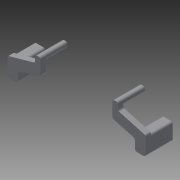
# Autodesk Inventor part: Solenoid Mount
Saved by Autodesk Inventor 2015 (Build 190159000, 159)
## iProperties
Created: 2016-09-23
Part Number: Solenoid Mount
Material: Generic
Document SubType Name: Modeling
Designer: James Yelland
Density: 1 g/cm^3
Appearance: Default
Author: James Yelland
Autodesk Inventor part; units mm, degrees
ref_plane "YZ Plane" through (0, 0, 0) normal (1, 0, 0) x (0, 1, 0)
ref_plane "XZ Plane" through (0, 0, 0) normal (0, 1, 0) x (-1, 0, 0)
ref_plane "XY Plane" through (0, 0, 0) normal (0, 0, 1) x (1, 0, 0)
sketch "Sketch1" plane through (0, 0, 0) normal (0, 1, 0) x (-1, 0, 0)
  line L0 (-54.0074, -78) -> (-54.0074, -71.5202)
  arc A0 (-52.5426, -69.5932) -> (-54.0074, -71.5202) centre (-52.0074, -71.5202) ccw
  arc A1 (-56.0074, -80) -> (-54.0074, -78) centre (-56.0074, -78) ccw
  line L1 (-54.0074, -78) -> (-54.0074, -71.5202)
  arc A2 (-52.5426, -69.5932) -> (-54.0074, -71.5202) centre (-52.0074, -71.5202) ccw
  arc A3 (-56.0074, -80) -> (-54.0074, -78) centre (-56.0074, -78) ccw
  line L2 (-54.0074, -78) -> (-54.0074, -71.5202)
  arc A4 (-52.5426, -69.5932) -> (-54.0074, -71.5202) centre (-52.0074, -71.5202) ccw
  arc A5 (-56.0074, -80) -> (-54.0074, -78) centre (-56.0074, -78) ccw
  line L3 (-62.0074, -80) -> (-56.0074, -80)
  line L4 (-64.0074, -78) -> (-64.0074, -64.2976)
  arc A6 (-62.5426, -62.3706) -> (-64.0074, -64.2976) centre (-62.0074, -64.2976) ccw
  arc A7 (-64.0074, -78) -> (-62.0074, -80) centre (-62.0074, -78) ccw
  line L5 (-52.5426, -69.5932) -> (-34.7368, -64.6478)
  line L6 (-33.272, -62.7207) -> (-33.272, -56.3381)
  line L7 (-33.272, -56.3381) -> (-33.272, -54)
  line L8 (-33.272, -54) -> (-33.272, -51)
  line L9 (-35.272, -49) -> (-36.272, -49)
  line L10 (-62.5426, -62.3706) -> (-39.7368, -56.0365)
  line L11 (-38.272, -54.1094) -> (-38.272, -51)
  arc A8 (-36.272, -49) -> (-38.272, -51) centre (-36.272, -51) ccw
  arc A9 (-33.272, -51) -> (-35.272, -49) centre (-35.272, -51) ccw
  arc A10 (-39.7368, -56.0365) -> (-38.272, -54.1094) centre (-40.272, -54.1094) ccw
  arc A11 (-34.7368, -64.6478) -> (-33.272, -62.7207) centre (-35.272, -62.7207) ccw
  line L12 (54.0074, -78) -> (54.0074, -71.5202)
  arc A12 (54.0074, -71.5202) -> (52.5426, -69.5932) centre (52.0074, -71.5202) ccw
  arc A13 (54.0074, -78) -> (56.0074, -80) centre (56.0074, -78) ccw
  line L13 (54.0074, -78) -> (54.0074, -71.5202)
  arc A14 (54.0074, -71.5202) -> (52.5426, -69.5932) centre (52.0074, -71.5202) ccw
  arc A15 (54.0074, -78) -> (56.0074, -80) centre (56.0074, -78) ccw
  line L14 (54.0074, -78) -> (54.0074, -71.5202)
  arc A16 (54.0074, -78) -> (56.0074, -80) centre (56.0074, -78) ccw
  arc A17 (54.0074, -71.5202) -> (52.5426, -69.5932) centre (52.0074, -71.5202) ccw
  line L15 (62.0074, -80) -> (56.0074, -80)
  line L16 (64.0074, -78) -> (64.0074, -64.2976)
  arc A18 (64.0074, -64.2976) -> (62.5426, -62.3706) centre (62.0074, -64.2976) ccw
  arc A19 (62.0074, -80) -> (64.0074, -78) centre (62.0074, -78) ccw
  line L17 (52.5426, -69.5932) -> (34.7368, -64.6478)
  line L18 (33.272, -62.7207) -> (33.272, -56.3381)
  line L19 (33.272, -56.3381) -> (33.272, -54)
  line L20 (33.272, -54) -> (33.272, -51)
  line L21 (35.272, -49) -> (36.272, -49)
  line L22 (62.5426, -62.3706) -> (39.7368, -56.0365)
  line L23 (38.272, -54.1094) -> (38.272, -51)
  arc A20 (38.272, -51) -> (36.272, -49) centre (36.272, -51) ccw
  arc A21 (35.272, -49) -> (33.272, -51) centre (35.272, -51) ccw
  arc A22 (38.272, -54.1094) -> (39.7368, -56.0365) centre (40.272, -54.1094) ccw
  arc A23 (33.272, -62.7207) -> (34.7368, -64.6478) centre (35.272, -62.7207) ccw
  point P0 (-33.272, -64.241)
  point P1 (-33.272, -49)
  point P2 (-38.272, -49)
  point P3 (33.272, -64.241)
  point P4 (33.272, -49)
  point P5 (38.272, -49)
  dimension "d11" = 2
  dimension "d29" = 20
  dimension "d30" = 5
  dimension "d31" = 5
  dimension "d32" = 2
  constraints: 48 end point, 48 point on circle, 24 centre point, 16 point on line, 13 tangent, 4 equal radius, 2 perpendicular, 1 vertical
  measures "d11" radius of A6
  measures "d29" distance of L5.start point (-33.272, -64.241)
  measures "d30" distance of L7.end point (-33.272, -49)
  measures "d31" distance of point (-33.272, -49) point (-38.272, -49)
  measures "d32" radius of A8
extrude "Extrusion1" add sketch "Sketch1" along normal blind 5
sketch "Sketch2" plane through (0, 5, 0) normal (0, 1, 0) x (1, 0, 0)
  line L0 (54.0074, 78) -> (54.0074, 71.5202) projected
  arc A0 (56.0074, 80) -> (54.0074, 78) centre (56.0074, 78) ccw projected
  line L1 (62.0074, 80) -> (56.0074, 80) projected
  arc A1 (64.0074, 78) -> (62.0074, 80) centre (62.0074, 78) ccw projected
  line L2 (64.0074, 64.2976) -> (64.0074, 78) projected
  line L3 (54.0074, 71.5202) -> (54.0074, 66.2976)
  line L4 (56.0074, 64.2976) -> (62.0074, 64.2976)
  line L5 (64.0074, 66.2976) -> (64.0074, 78)
  arc A2 (62.0074, 64.2976) -> (64.0074, 66.2976) centre (62.0074, 66.2976) ccw
  arc A3 (54.0074, 66.2976) -> (56.0074, 64.2976) centre (56.0074, 66.2976) ccw
  line L6 (0, 44.0707) -> (0, 74.7601)
  line L7 (-54.0074, 78) -> (-54.0074, 71.5202)
  arc A4 (-54.0074, 78) -> (-56.0074, 80) centre (-56.0074, 78) ccw
  line L8 (-62.0074, 80) -> (-56.0074, 80)
  arc A5 (-62.0074, 80) -> (-64.0074, 78) centre (-62.0074, 78) ccw
  line L9 (-64.0074, 64.2976) -> (-64.0074, 78)
  line L10 (-54.0074, 71.5202) -> (-54.0074, 66.2976)
  line L11 (-56.0074, 64.2976) -> (-62.0074, 64.2976)
  line L12 (-64.0074, 66.2976) -> (-64.0074, 78)
  arc A6 (-64.0074, 66.2976) -> (-62.0074, 64.2976) centre (-62.0074, 66.2976) ccw
  arc A7 (-56.0074, 64.2976) -> (-54.0074, 66.2976) centre (-56.0074, 66.2976) ccw
  line L13 (38.272, 51) -> (38.272, 54.1094) projected
  arc A8 (36.272, 49) -> (38.272, 51) centre (36.272, 51) ccw projected
  line L14 (35.272, 49) -> (36.272, 49) projected
  arc A9 (33.272, 51) -> (35.272, 49) centre (35.272, 51) ccw projected
  line L15 (33.272, 62.7207) -> (33.272, 51) projected
  line L16 (36.272, 49) -> (35.272, 49) projected
  line L17 (35.772, 49) -> (35.772, 54)
  line L18 (35.772, 54) -> (35.272, 54)
  line L19 (33.272, 51) -> (33.272, 62.7207) projected
  line L20 (35.772, 54) -> (36.272, 54)
  line L21 (38.272, 54.1094) -> (38.272, 51) projected
  line L22 (-38.272, 51) -> (-38.272, 52)
  arc A10 (-38.272, 51) -> (-36.272, 49) centre (-36.272, 51) ccw
  line L23 (-35.272, 49) -> (-36.272, 49)
  arc A11 (-35.272, 49) -> (-33.272, 51) centre (-35.272, 51) ccw
  line L24 (-33.272, 52) -> (-33.272, 51)
  line L25 (-36.272, 49) -> (-35.272, 49)
  line L26 (-35.772, 49) -> (-35.772, 54)
  line L27 (-35.772, 54) -> (-35.272, 54)
  line L28 (-33.272, 51) -> (-33.272, 62.7207)
  line L29 (-35.772, 54) -> (-36.272, 54)
  line L30 (-38.272, 54.1094) -> (-38.272, 51)
  line L31 (38.272, 52) -> (38.272, 51)
  line L32 (33.272, 52) -> (33.272, 51)
  arc A12 (-33.272, 52) -> (-35.272, 54) centre (-35.272, 52) ccw
  arc A13 (-36.272, 54) -> (-38.272, 52) centre (-36.272, 52) ccw
  arc A14 (38.272, 52) -> (36.272, 54) centre (36.272, 52) ccw
  arc A15 (35.272, 54) -> (33.272, 52) centre (35.272, 52) ccw
  point P0 (0, 0)
  point P1 (33.272, 54)
  point P2 (38.272, 54)
  point P3 (-33.272, 54)
  point P4 (-38.272, 54)
  dimension "d19" = 2
  dimension "d33" = 5
  dimension "d34" = 2
  constraints: 48 end point, 26 symmetric about line, 24 point on circle, 16 point on line, 12 centre point, 12 tangent, 4 equal radius, 4 vertical, 2 collinear, 2 perpendicular, 1 horizontal, 1 midpoint, 6 other
  measures "d19" radius of A2
  measures "d33" distance of L17.start L17.end
  measures "d34" radius of A12
extrude "Extrusion2" add sketch "Sketch2" along normal blind 20
body "Solid1"
